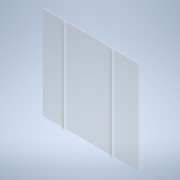
# Autodesk Inventor part: poly carbonate plate
Saved by Autodesk Inventor 2021 (Build 250183000, 183)
## iProperties
Created: 2022-05-21
Part Number: poly carbonate plate
Material: Polycarbonate, Clear
Document SubType Name: Modeling
Designer: techv
Mass: 126.54 g
Surface Area: 725.5 cm^2
Volume: 105.45 cm^3
Density: 1.2 g/cm^3
Appearance: Polycarbonate - Clear
Author: techv
Autodesk Inventor part; units mm, degrees
ref_plane "YZ Plane" through (0, 0, 0) normal (1, 0, 0) x (0, 1, 0)
ref_plane "XZ Plane" through (0, 0, 0) normal (0, 1, 0) x (-1, 0, 0)
ref_plane "XY Plane" through (0, 0, 0) normal (0, 0, 1) x (1, 0, 0)
sketch "Sketch1" plane through (0, 0, 0) normal (0, 0, 1) x (1, 0, 0)
  line L0 (-95, -92.5) -> (95, -92.5)
  line L1 (95, -92.5) -> (95, 92.5)
  line L2 (95, 92.5) -> (-95, 92.5)
  line L3 (-95, 92.5) -> (-95, -92.5)
  line L4 (-95, -92.5) -> (95, 92.5) construction
  line L5 (95, -92.5) -> (-95, 92.5) construction
  point P0 (0, 0)
  dimension "d0" = 190
  dimension "d1" = 185
  constraints: 12 end point, 2 midpoint, 2 parallel, 1 horizontal, 1 perpendicular
  measures "d0" distance of L1.end L2.end
  measures "d1" distance of L2.end L0.start
extrude "Extrusion1" add sketch "Sketch1" along normal blind 3
sketch "Sketch2" plane through (-95, 92.5, 0) normal (0, 1, 0) x (1, 0, 0)
  line L0 (190, -3) -> (0, -3) projected
  line L1 (142.5, -3) -> (137.5, -3)
  line L2 (137.5, -3) -> (137.5, -8)
  line L3 (137.5, -8) -> (142.5, -8)
  line L4 (142.5, -8) -> (142.5, -3)
  line L5 (47.5, -3) -> (42.5, -3)
  line L6 (42.5, -3) -> (42.5, -8)
  line L7 (42.5, -8) -> (47.5, -8)
  line L8 (47.5, -8) -> (47.5, -3)
  point P0 (95, 0)
  dimension "d4" = 5
  dimension "d5" = 5
  dimension "d6" = 5
  dimension "d7" = 5
  dimension "d8" = 47.5
  dimension "d9" = 142.5
  constraints: 16 end point, 4 parallel, 2 horizontal, 2 perpendicular, 2 point on line
  measures "d4" distance of L3.end L2.end
  measures "d5" distance of L2.end L1.end
  measures "d6" distance of L7.end L6.end
  measures "d7" distance of L6.end L5.end
  measures "d8" horizontal distance of L3.end L0.start
  measures "d9" horizontal distance of L0.start L7.end
extrude "Extrusion2" add sketch "Sketch2" against normal up to surface (185 mm away)
body "Solid1"
